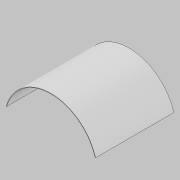
# Autodesk Inventor part: cover_shell1
Saved by Autodesk Inventor 2021 (Build 250183000, 183)
## iProperties
Created: 2021-05-06
Part Number: cover_shell1
Material: Generic
Document SubType Name: Modeling
Designer: Watchdog
Density: 1 g/cm^3
Appearance: Default
Author: Watchdog
Autodesk Inventor part; units mm, degrees
ref_plane "YZ Plane" through (0, 0, 0) normal (1, 0, 0) x (0, 1, 0)
ref_plane "XZ Plane" through (0, 0, 0) normal (0, 1, 0) x (-1, 0, 0)
ref_plane "XY Plane" through (0, 0, 0) normal (0, 0, 1) x (1, 0, 0)
sketch "Sketch2" plane through (0, 0, 0) normal (0, 0, 1) x (1, 0, 0)
  arc A0 (800, 0) -> (-800, 0) centre (0, -233.3333) ccw
  arc A1 (790, 0) -> (-790, 0) centre (0, -233.3333) ccw
  line L0 (541.3488, 0) -> (790, 0)
  line L1 (-790, 0) -> (-800, 0)
  line L2 (800, 0) -> (790, 0)
  line L3 (-790, 0) -> (-800, 0)
  point P0 (0, 0)
  point P1 (0, 600)
  dimension "d12" = 1600
  dimension "d13" = 600
  dimension "d16" = 0
  dimension "d17" = 0
  dimension "d18" = 0
  dimension "d19" = 0
  dimension "d20" = 0
  dimension "d21" = 0
  dimension "d23" = 10
  constraints: 8 end point, 5 point on circle, 2 centre point, 1 coincident, 1 horizontal
  measures "d12" distance of L1.end L2.start
  measures "d13" distance of point (0, 0) point (0, 600)
  measures "d16" horizontal distance of point (0, 0) A0.centre
  measures "d17" horizontal distance of point (0, 0) point (0, 600)
  measures "d18" vertical distance of point (0, 0) L2.start
  measures "d19" vertical distance of point (0, 0) L1.end
  measures "d20" vertical distance of point (0, 0) L0.end
  measures "d21" vertical distance of point (0, 0) L1.start
  measures "d23" distance of L2.start L0.end
extrude "shell" add sketch "Sketch2" along normal blind 1400
equation "\"d12\" = cover_length_main"
equation "\"d13\" = cover_height_main"
equation "\"d23\" = cover_shell_thickness"
equation "\"d14\" = cover_width_main"
equation "\"rack_tooth_thickness\" = 5"
equation "\"rack_tooth_addendum\" = 5"
equation "\"rack_tooth_dedendum\" = 5"
equation "\"cover_width_main\" = 1400"
equation "\"cover_height_main\" = 600"
equation "\"cover_length_main\" = 1600"
equation "\"cover_shell_thickness\" = 10"
body "Solid2"
